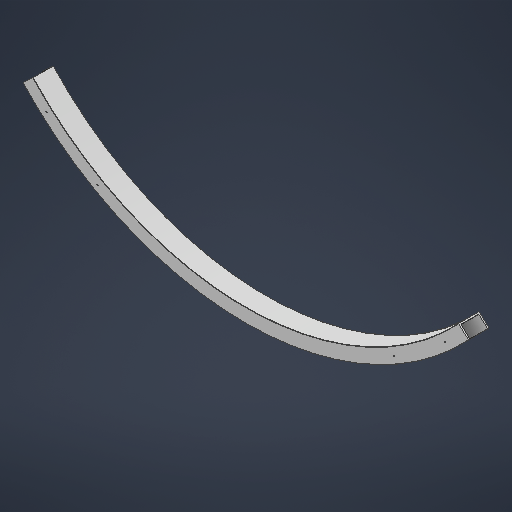
# Autodesk Inventor part: Sled
Saved by Autodesk Inventor 2026.1 (Build 301233020, 233B)
## iProperties
Created: 2025-11-03
Part Number: Sled
Material: Generic
Document SubType Name: Modeling
Designer: Study
Density: 1 g/cm^3
Appearance: Default
Author: Study
Autodesk Inventor part; units mm, degrees
ref_plane "YZ Plane" through (0, 0, 0) normal (1, 0, 0) x (0, 1, 0)
ref_plane "XZ Plane" through (0, 0, 0) normal (0, 1, 0) x (-1, 0, 0)
ref_plane "XY Plane" through (0, 0, 0) normal (0, 0, 1) x (1, 0, 0)
sketch "Sketch1" plane through (0, 0, 0) normal (1, 0, 0) x (0, 1, 0)
  line L0 (0, 0) -> (0, -75)
  line L1 (0, -75) -> (-100, -75)
  line L2 (-100, -75) -> (-100, -65)
  line L3 (-100, -65) -> (-10, -65)
  line L4 (-10, -65) -> (-10, 0)
  line L5 (0, 0) -> (0, 75)
  line L6 (0, 75) -> (-100, 75)
  line L7 (-100, 75) -> (-100, 65)
  line L8 (-100, 65) -> (-10, 65)
  line L9 (-10, 65) -> (-10, 0)
  dimension "d1" = 75
  dimension "d2" = 100
  dimension "d3" = 10
  dimension "d4" = 10
  dimension "d5" = 10
  constraints: 20 end point, 2 perpendicular, 1 parallel, 1 vertical
  measures "d1" distance of L0.start L0.end
  measures "d2" distance of L0.end L1.end
  measures "d3" distance of L0.start L4.end
  measures "d4" distance from line of L1 L3.end
  measures "d5" distance of L1.end L2.end
sketch "Sketch2" plane through (0, 0, 0) normal (1, 0, 0) x (0, 1, 0)
  point P0 (0, 0)
  point P1 (2125, 0)
sketch "Sketch3" plane through (0, 0, 0) normal (1, 0, 0) x (0, 1, 0)
  line L0 (0, 0) -> (2125, 0) construction
  line L1 (2125, 0) -> (2125, -62.9118) construction
  dimension "d9" = 2125
  constraints: 4 end point, 1 horizontal, 1 perpendicular
  measures "d9" distance of L0.start L0.end
revolve "Revolution1" add sketch "Sketch1" angle 47 about axis through (0, 2125, 0) along (0, 0, 1)
sketch "Sketch5" plane through (0, -100, 75) normal (0, 0, 1) x (1, 0, 0)
  arc A0 (0, 90) -> (1561.4402, 768.9335) centre (0, 2225) ccw projected
  line L0 (0, 90) -> (0, 2225) construction
  line L1 (0, 0) -> (0, 100) projected
  arc A1 (0, 50) -> (867.2792, 230.3943) centre (0, 2225) ccw construction
  arc A2 (0, 50) -> (1455.3591, 608.66) centre (0, 2225) ccw construction
  line L2 (0, 100) -> (0, 0) projected
  point P0 (0, 50)
  point P1 (0, 50)
  dimension "d19" = 42
  dimension "d20" = 23.5
  constraints: 4 point on circle, 3 midpoint, 2 centre point, 2 end point, 1 coincident, 1 vertical
hole "Hole2" at (1455.3591, 508.66, 75) direction (0, 0, -1) diameter 10 end through all
mirror "Mirror1" about plane through (0, 0, 0) normal (1, 0, 0)
fillet "Fillet1" radius 2 1 edges at (0, 0, 75)
fillet "Fillet2" radius 1 1 edges at (0, -100, 75)
fillet "Fillet3" radius 1 1 edges at (0, -100, 65)
fillet "Fillet4" radius 1 1 edges at (0, -100, -65)
fillet "Fillet5" radius 1 1 edges at (0, -100, -75)
fillet "Fillet6" radius 2 1 edges at (0, 0, -75)
fillet "Fillet7" radius 2 1 edges at (0, -10, 65)
fillet "Fillet8" radius 2 1 edges at (0, -10, -65)
sketch "Sketch7" plane through (0, 0, 0) normal (0, 0, 1) x (1, 0, 0)
  arc A0 (-1626.5306, 608.2356) -> (1626.5306, 608.2356) centre (0, 2125) ccw projected
  line L0 (-1555.5893, 674.3895) -> (-1554.1266, 675.7535) projected
  circle A1 centre (0, 2125) radius 2125
  circle A2 centre (-1455.3591, 508.66) radius 5 projected
  line L1 (-1455.3591, 508.66) -> (-1594.2776, -279.1862)
  line L2 (-1455.3591, 508.66) -> (-655.3591, 508.66) construction
  line L3 (-1594.2776, -279.1862) -> (-661.0542, -279.1862) construction
  line L4 (-1594.2776, -279.1862) -> (-1081.6252, 233.4662)
  line L5 (-1594.2776, -279.1862) -> (-869.2776, -279.1862) construction
  circle A3 centre (-1081.6252, 233.4662) radius 5
  line L6 (-1618.8978, -274.845) -> (-1479.9793, 513.0012)
  line L7 (-1479.9793, 513.0012) -> (-1430.7389, 504.3188)
  line L8 (-1430.7389, 504.3188) -> (-1569.6574, -283.5274)
  line L9 (-1569.6574, -283.5274) -> (-1618.8978, -274.845)
  line L10 (-1618.8978, -274.845) -> (-1430.7389, 504.3188) construction
  line L11 (-1479.9793, 513.0012) -> (-1569.6574, -283.5274) construction
  line L12 (-1099.3029, 251.1439) -> (-1611.9553, -261.5085)
  line L13 (-1611.9553, -261.5085) -> (-1576.5999, -296.8639)
  line L14 (-1576.5999, -296.8639) -> (-1063.9475, 215.7885)
  line L15 (-1063.9475, 215.7885) -> (-1099.3029, 251.1439)
  line L16 (-1099.3029, 251.1439) -> (-1576.5999, -296.8639) construction
  line L17 (-1611.9553, -261.5085) -> (-1063.9475, 215.7885) construction
  line L18 (-1555.8889, -205.4421) -> (-1520.5335, -240.7975) construction
  line L19 (-1563.4575, -248.3661) -> (-1545.7799, -266.0438) construction
  point P0 (0, 0)
  point P1 (0, -99)
  point P2 (-1554.858, 675.0715)
  point P3 (0, -99)
  point P4 (-1524.8183, 114.7369)
  point P5 (-1337.9514, -22.86)
  point P6 (-1554.6187, -257.205)
  dimension "d44" = 774.0715
  dimension "d45" = 800
  dimension "d46" = 100
  dimension "d49" = 180.1862
  dimension "d50" = 725
  dimension "d51" = 45
  dimension "d52" = 10
  dimension "d55" = 50
  dimension "d56" = 50
  dimension "d57" = 35.7037
  dimension "d58" = 43.5862
  dimension "d59" = 79.2899
  constraints: 38 end point, 8 midpoint, 6 parallel, 6 point on line, 4 perpendicular, 3 horizontal, 2 centre point, 2 coincident, 2 equal length, 2 point on circle
  measures "d44" vertical distance of point (0, -99) point (-1554.858, 675.071)
  measures "d45" distance of L1.start L1.end
  measures "d46" angle of L1 L2
  measures "d49" vertical distance of L1.end point (0, -99)
  measures "d50" distance of L1.end L4.end
  measures "d51" angle of L5 L4
  measures "d52" diameter of A3
  measures "d55" distance of L6.end L7.end
  measures "d56" distance of L13.end L12.end
  measures "d57" distance from line of point (-1554.619, -257.205) L18
  measures "d58" distance between parallel lines of L13 L19
  measures "d59" distance between parallel lines of L18 L13
extrude "Extrusion1" cut sketch "Sketch7" along normal mid plane 150 contours A3 L15 L4 | L4 L15 A3 | A3 L15
mirror "Mirror2" about plane through (0, 0, 0) normal (1, 0, 0) of "Extrusion1"
body "Solid1"
